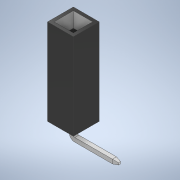
# Autodesk Inventor part: FemaleHederPin_90
Saved by Autodesk Inventor 2021 (Build 250183000, 183)
## iProperties
Created: 2020-01-02
Part Number: FemaleHederPin_90
Material: Generic
Document SubType Name: Modeling
Designer: ermoz
Density: 1 g/cm^3
Appearance: Default
Mass: 0.0534802 g
Surface Area: 1.12055 cm^2
Volume: 0.0534802 cm^3
Author: ermoz
Autodesk Inventor part; units mm, degrees
ref_plane "YZ Plane" through (0, 0, 0) normal (1, 0, 0) x (0, 1, 0)
ref_plane "XZ Plane" through (0, 0, 0) normal (0, 1, 0) x (-1, 0, 0)
ref_plane "XY Plane" through (0, 0, 0) normal (0, 0, 1) x (1, 0, 0)
sketch "Sketch1" plane through (0, 0, 0) normal (0, 1, 0) x (-1, 0, 0)
  line L0 (-1.27, 1.27) -> (1.27, 1.27)
  line L1 (1.27, 1.27) -> (1.27, -1.27)
  line L2 (1.27, -1.27) -> (-1.27, -1.27)
  line L3 (-1.27, -1.27) -> (-1.27, 1.27)
  line L4 (-1.27, 1.27) -> (1.27, -1.27) construction
  line L5 (1.27, 1.27) -> (-1.27, -1.27) construction
  point P0 (0, 0)
  dimension "d0" = 2.54
  dimension "d1" = 2.54
  constraints: 12 end point, 2 midpoint, 2 parallel, 1 horizontal, 1 perpendicular
  measures "d0" distance of L1.end L2.end
  measures "d1" distance of L0.end L1.end
extrude "Extrusion1" add sketch "Sketch1" along normal blind 8.5
sketch "Sketch2" plane through (0, 8.5, 0) normal (0, 1, 0) x (1, 0, 0)
  line L0 (0.2, -0.2) -> (-0.2, -0.2)
  line L1 (-0.2, -0.2) -> (-0.2, 0.2)
  line L2 (-0.2, 0.2) -> (0.2, 0.2)
  line L3 (0.2, 0.2) -> (0.2, -0.2)
  line L4 (0.2, -0.2) -> (-0.2, 0.2) construction
  line L5 (-0.2, -0.2) -> (0.2, 0.2) construction
  point P0 (0, 0)
  dimension "d4" = 0.4
  dimension "d5" = 0.4
  constraints: 12 end point, 2 midpoint, 2 parallel, 1 horizontal, 1 perpendicular
  measures "d4" distance of L1.end L2.end
  measures "d5" distance of L0.end L1.end
extrude "Extrusion2" cut sketch "Sketch2" against normal blind 5
chamfer "Chamfer1" distance 0.75 angle 45 4 edges at (0, 8.5, 0.2) (-0.2, 8.5, 0) (0, 8.5, -0.2) (0.2, 8.5, 0)
sketch "Sketch3" plane through (0, 0, 0) normal (0, -1, 0) x (1, 0, 0)
  line L0 (-0.2, 0.2) -> (0.2, 0.2)
  line L1 (0.2, 0.2) -> (0.2, -0.2)
  line L2 (0.2, -0.2) -> (-0.2, -0.2)
  line L3 (-0.2, -0.2) -> (-0.2, 0.2)
  line L4 (-0.2, 0.2) -> (0.2, -0.2) construction
  line L5 (0.2, 0.2) -> (-0.2, -0.2) construction
  point P0 (0, 0)
  dimension "d11" = 0.4
  dimension "d12" = 0.4
  constraints: 12 end point, 2 midpoint, 2 parallel, 1 horizontal, 1 perpendicular
  measures "d11" distance of L1.end L2.end
  measures "d12" distance of L0.end L1.end
extrude "Extrusion3" add sketch "Sketch3" along normal blind 1.5
sketch "Sketch4" plane through (-0.2, 0, 0.2) normal (0, 0, 1) x (1, 0, 0)
  line L0 (0, -1.5) -> (4.75, -1.5)
  line L1 (4.75, -1.5) -> (4.75, -1.1)
  line L2 (4.75, -1.1) -> (0, -1.1)
  line L3 (0, -1.1) -> (0, -1.5)
  point P0 (0.2, 0)
  dimension "d27" = 0.4
  dimension "d28" = 4.75
  constraints: 8 end point, 2 parallel, 1 horizontal, 1 perpendicular
  measures "d27" distance of L0.end L1.end
  measures "d28" distance of L0.start L0.end
extrude "Extrusion4" add sketch "Sketch4" against normal up to surface (0.4 mm away)
fillet "Fillet1" radius 0.5 1 edges at (-0.2, -1.5, 0)
fillet "Fillet2" radius 0.15 1 edges at (0.2, -1.1, 0)
chamfer "Chamfer6" distance 0.5 distance2 0.1 1 edges at (4.55, -1.3, 0.2) measured on face at (1.7333, -1.3667, 0.2)
chamfer "Chamfer7" distance 0.5 distance2 0.1 1 edges at (4.55, -1.1, -0.05) measured on face at (2.9833, -1.1, -0.0667)
chamfer "Chamfer8" distance 0.1 distance2 0.5 1 edges at (4.55, -1.35, -0.2) measured on face at (4.55, -1.4, 0)
chamfer "Chamfer9" distance 0.1 distance2 0.5 1 edges at (4.55, -1.5, 0) measured on face at (4.55, -1.4, 0.0333)
body "Solid1"
